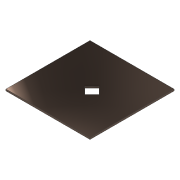
# Autodesk Inventor part: wer
Saved by Autodesk Inventor 2021 (Build 250183000, 183)
## iProperties
Created: 2021-07-25
Part Number: wer
Material: Generic
Document SubType Name: Modeling
Designer: Shaheen Khan
Density: 1 g/cm^3
Appearance: Default
Author: Shaheen Khan
Autodesk Inventor part; units mm, degrees
ref_plane "YZ Plane" through (0, 0, 0) normal (1, 0, 0) x (0, 1, 0)
ref_plane "XZ Plane" through (0, 0, 0) normal (0, 1, 0) x (-1, 0, 0)
ref_plane "XY Plane" through (0, 0, 0) normal (0, 0, 1) x (1, 0, 0)
sketch "Sketch1" plane through (0, 0, 0) normal (0, 1, 0) x (-1, 0, 0)
  line L0 (-250, 250) -> (250, 250)
  line L1 (250, 250) -> (250, -250)
  line L2 (250, -250) -> (-250, -250)
  line L3 (-250, -250) -> (-250, 250)
  line L4 (-250, 250) -> (250, -250) construction
  line L5 (250, 250) -> (-250, -250) construction
  line L6 (-12.4264, 42.4417) -> (30, 0.0153)
  line L7 (30, 0.0153) -> (-12.4264, -42.4112)
  line L8 (-12.4264, -42.4112) -> (-54.8528, 0.0153)
  line L9 (-54.8528, 0.0153) -> (-12.4264, 42.4417)
  point P0 (0, 0)
  dimension "d0" = 500
  dimension "d1" = 60
  dimension "d2" = 30
  dimension "d3" = 54.8528
  constraints: 20 end point, 7 perpendicular, 2 midpoint, 2 parallel, 1 horizontal
  measures "d0" distance of L0.end L1.end
  measures "d1" distance of L6.start L6.end
  measures "d2" distance of point (0, 0) L6.end
  measures "d3" distance of L8.end point (0, 0)
extrude "Extrusion1" add sketch "Sketch1" along normal blind 10
body "Solid1"
